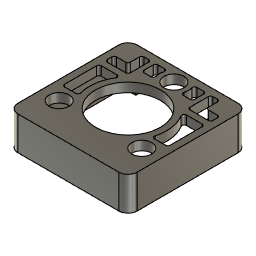
Laser Shroud (Autodesk Fusion 360 design; units mm, degrees)
Autodesk Fusion 360 part; units mm, degrees
sketch "Sketch1" plane through (0, 0, 0) normal (0, 0, 1) x (1, 0, 0) in component "Laser Shroud Mount"
  line L0 (0, 0) -> (39, 0)
  line L1 (39, 0) -> (39, 39)
  line L2 (39, 39) -> (0, 39)
  line L3 (0, 39) -> (0, 0)
  dimension "d1" = 39
  dimension "d2" = 39
  constraint horizontal L0
  constraint vertical L1
  constraint horizontal L2
  constraint vertical L3
  constraint coincident L0.start L3.end
  measures "d1" distance of L0.start L0.end
  measures "d2" distance of L0.start L2.end
extrude "Extrude1" add sketch "Sketch1" along normal blind 3 in component "Laser Shroud Mount"
sketch "Sketch2" plane through (0, 0, 3) normal (0, 0, 1) x (-1, 0, 0) in component "Laser Shroud Mount"
  line L0 (0, -39) -> (0, 0)
  line L1 (0, 0) -> (-39, 0)
  line L2 (-39, 0) -> (-39, -39)
  line L3 (-39, -39) -> (0, -39)
  line L4 (-19.5, -39) -> (-19.5, 0) construction
  line L5 (0, -19.5) -> (-39, -19.5) construction
  circle A0 centre (-19.5, -19.5) radius 10.6
  line L6 (-35, -35) -> (-4, -35) construction
  line L7 (-4, -35) -> (-4, -4) construction
  line L8 (-4, -4) -> (-35, -4) construction
  line L9 (-35, -4) -> (-35, -35) construction
  line L10 (-35, -35) -> (-4, -4) construction
  line L11 (-4, -35) -> (-35, -4) construction
  circle A1 centre (-4, -35) radius 1.75
  circle A2 centre (-35, -35) radius 1.75
  circle A3 centre (-4, -4) radius 1.75
  circle A4 centre (-35, -4) radius 1.75
  point P0 (-19.5, -19.5)
  dimension "d5" = 21.2
  dimension "d6" = 31
  dimension "d7" = 31
  dimension "d8" = 3.5
  dimension "d9" = 3.5
  dimension "d10" = 3.5
  dimension "d11" = 3.5
  constraint midpoint L3 L4.start
  constraint midpoint L1 L4.end
  constraint midpoint L0 L5.start
  constraint midpoint L2 L5.end
  constraint midpoint L5 P0
  constraint horizontal L6
  constraint perpendicular L6 L7
  constraint parallel L6 L8
  constraint parallel L7 L9
  constraint coincident L10 P0
  constraint coincident L11 P0
  constraint coincident P0 A0.centre
  constraint coincident L6.end L7.start
  constraint coincident L6.start L9.end
  constraint coincident L7.end L8.start
  constraint coincident L8.end L9.start
  measures "d5" diameter of A0
  measures "d6" distance of L7.end L8.end
  measures "d7" distance of L6.end L7.end
  measures "d8" diameter of A1
  measures "d9" diameter of A2
  measures "d10" diameter of A3
  measures "d11" diameter of A4
extrude "Extrude2" cut sketch "Sketch2" against normal up to surface (3 mm away) contours A0 in component "Laser Shroud Mount"
sketch "Sketch3" plane through (0, 0, 3) normal (0, 0, 1) x (-1, 0, 0) in component "Laser Shroud Mount"
  circle A0 centre (-19.5, -19.5) radius 10.6
  line L0 (0, -39) -> (0, 0)
  line L1 (0, 0) -> (-39, 0)
  line L2 (-39, 0) -> (-39, -39)
  line L3 (-39, -39) -> (0, -39)
  line L4 (-19.5, -39) -> (-19.5, 0) construction
  line L5 (0, -34.5) -> (-39, -34.5) construction
  circle A1 centre (-19.5, -34.5) radius 3.25
  line L6 (0, -10.5) -> (-39, -10.5) construction
  line L7 (-6, -39) -> (-6, 0) construction
  circle A2 centre (-6, -10.5) radius 3.25
  line L8 (-33, -39) -> (-33, 0) construction
  circle A3 centre (-33, -10.5) radius 3.25
  dimension "d14" = 4.5
  dimension "d15" = 6.5
  dimension "d16" = 6.5
  dimension "d18" = 10.5
  dimension "d19" = 6
  dimension "d21" = 6
  dimension "d22" = 6.5
  constraint midpoint L3 L4.start
  constraint midpoint L1 L4.end
  constraint coincident L0 L5.start
  constraint coincident L2 L5.end
  constraint perpendicular L2 L5
  constraint midpoint L5 A1.centre
  constraint coincident L0 L6.start
  constraint coincident L2 L6.end
  constraint perpendicular L2 L6
  constraint coincident L1 L7.end
  constraint perpendicular L1 L7
  constraint coincident L7 A2.centre
  constraint coincident L6 A2.centre
  constraint coincident L3 L8.start
  constraint coincident L1 L8.end
  constraint perpendicular L1 L8
  constraint coincident L8 A3.centre
  constraint coincident L6 A3.centre
  measures "d14" distance of L3 L5
  measures "d15" diameter of A1
  measures "d16" diameter of A2
  measures "d18" distance of L1 L6
  measures "d19" distance of L0 L7
  measures "d21" distance of L2 L8
  measures "d22" diameter of A3
extrude "Extrude3" cut sketch "Sketch3" against normal blind 3.2 contours A1 | A2 | A3 in component "Laser Shroud Mount"
sketch "Sketch4" plane through (0, 0, 3) normal (0, 0, 1) x (-1, 0, 0) in component "Laser Shroud Mount"
  circle A0 centre (-19.5, -34.5) radius 3.25 construction
  circle A1 centre (-6, -10.5) radius 3.25
  circle A2 centre (-33, -10.5) radius 3.25
  circle A3 centre (-19.5, -19.5) radius 10.6
  line L0 (0, -39) -> (0, 0)
  line L1 (0, 0) -> (-39, 0)
  line L2 (-39, 0) -> (-39, -39)
  line L3 (-39, -39) -> (0, -39)
  line L4 (0, -36.75) -> (-39, -36.75) construction
  line L5 (-6.75, -39) -> (-6.75, 0) construction
  line L6 (-32.25, -39) -> (-32.25, 0) construction
  line L7 (0, -32.25) -> (-39, -32.25) construction
  line L8 (-6.75, -36.75) -> (-6.75, -32.25)
  line L9 (-2.25, -39) -> (-2.25, 0) construction
  line L10 (-6.75, -32.25) -> (-2.25, -32.25)
  line L11 (-2.25, -32.25) -> (-2.25, -29.25)
  line L12 (0, -19.5) -> (-39, -19.5) construction
  line L13 (-19.5, -39) -> (-19.5, 0) construction
  line L14 (-6.75, -36.75) -> (-9.75, -36.75)
  line L15 (-2.25, -29.25) -> (-9.75, -29.25)
  line L16 (-9.75, -29.25) -> (-9.75, -36.75)
  line L17 (-11.25, -36.75) -> (-11.25, -32.25)
  line L18 (-11.25, -36.75) -> (-15.3167, -36.75)
  line L19 (-11.25, -32.25) -> (-15.3167, -32.25)
  line L20 (-2.25, -27.25) -> (-9.5653, -27.25)
  line L21 (-2.25, -15.25) -> (-7.6384, -15.25)
  line L22 (-2.25, -27.25) -> (-2.25, -15.25)
  line L23 (0, -2) -> (-39, -2) construction
  arc A4 (-9.5653, -27.25) -> (-7.6384, -15.25) centre (-19.5, -19.5) ccw
  arc A5 (-15.3167, -36.75) -> (-15.3167, -32.25) centre (-19.5, -34.5) ccw
  arc A6 (-31.3616, -15.25) -> (-29.4347, -27.25) centre (-19.5, -19.5) ccw
  line L24 (-36.75, -15.25) -> (-31.3616, -15.25)
  line L25 (-36.75, -27.25) -> (-36.75, -15.25)
  line L26 (-36.75, -27.25) -> (-29.4347, -27.25)
  line L27 (-36.75, -29.25) -> (-29.25, -29.25)
  line L28 (-36.75, -32.25) -> (-36.75, -29.25)
  line L29 (-29.25, -29.25) -> (-29.25, -36.75)
  line L30 (-32.25, -32.25) -> (-36.75, -32.25)
  line L31 (-32.25, -36.75) -> (-32.25, -32.25)
  line L32 (-32.25, -36.75) -> (-29.25, -36.75)
  line L33 (-27.75, -36.75) -> (-27.75, -32.25)
  arc A7 (-23.6833, -32.25) -> (-23.6833, -36.75) centre (-19.5, -34.5) ccw
  line L34 (-27.75, -32.25) -> (-23.6833, -32.25)
  line L35 (-27.75, -36.75) -> (-23.6833, -36.75)
  dimension "d25" = 2.25
  dimension "d26" = 6.75
  dimension "d27" = 6.75
  dimension "d28" = 6.75
  dimension "d29" = 3
  dimension "d34" = 3
  dimension "d35" = 1.5
  dimension "d36" = 2
  dimension "d37" = 12
  dimension "d38" = 2
  constraint coincident L0 L4.start
  constraint coincident L2 L4.end
  constraint perpendicular L2 L4
  constraint coincident L3 L5.start
  constraint coincident L1 L5.end
  constraint perpendicular L1 L5
  constraint coincident L3 L6.start
  constraint coincident L1 L6.end
  constraint perpendicular L1 L6
  constraint coincident L0 L7.start
  constraint coincident L2 L7.end
  constraint perpendicular L2 L7
  constraint coincident L4 L8.start
  constraint coincident L5 L8.start
  constraint coincident L5 L8.end
  constraint coincident L7 L8.end
  constraint perpendicular L7 L8
  constraint coincident L3 L9.start
  constraint coincident L1 L9.end
  constraint perpendicular L1 L9
  constraint coincident L9 L10.end
  constraint coincident L7 L10.end
  constraint perpendicular L7 L11
  constraint midpoint L0 L12.start
  constraint midpoint L2 L12.end
  constraint midpoint L3 L13.start
  constraint midpoint L1 L13.end
  constraint perpendicular L8 L14
  constraint perpendicular L11 L15
  constraint perpendicular L4 L16
  constraint coincident L4 L17.start
  constraint coincident L7 L17.end
  constraint perpendicular L7 L17
  constraint coincident L4 L18.end
  constraint coincident L7 L19.end
  constraint coincident L9 L20.start
  constraint perpendicular L9 L20
  constraint coincident L9 L21.start
  constraint perpendicular L5 L21
  constraint coincident L0 L23.start
  constraint coincident L2 L23.end
  constraint perpendicular L2 L23
  constraint concentric A3 A4
  constraint symmetric L8.start L13 L31.start
  constraint symmetric L8.end L13 L30.start
  constraint symmetric L10.end L13 L28.start
  constraint symmetric L11.end L13 L27.start
  constraint symmetric L13 L14.end L29.end
  constraint symmetric L13 L15.end L27.end
  constraint symmetric L13 L17.start L33.start
  constraint symmetric L13 L17.end L33.end
  constraint symmetric L13 L18.end A7.end
  constraint symmetric L13 L19.end A7.start
  constraint symmetric L13 L20.start L25.start
  constraint symmetric L13 L20.end A6.end
  constraint symmetric L13 L21.start L24.start
  constraint symmetric L13 L21.end A6.start
  constraint symmetric L13 A4 A6
  constraint symmetric L13 A5 A7
  measures "d25" distance of L3 L4
  measures "d26" distance of L0 L5
  measures "d27" distance of L2 L6
  measures "d28" distance of L3 L7
  measures "d29" distance of L10.end L11.end
  measures "d34" distance of L8.start L14.end
  measures "d35" distance of L16 L17
  measures "d36" distance of L15 L20
  measures "d37" distance of L20 L21
  measures "d38" distance of L1 L23
extrude "Extrude4" cut sketch "Sketch4" against normal up to surface (3 mm away) contours L8 L10 L11 L14 L15 L16 | L17 L18 L19 A5 | L20 L21 L22 A4 | A6 L24 L25 L26 | L27 L28 L29 L30 L31 L32 | L33 A7 L34 L35 in component "Laser Shroud Mount"
fillet "Fillet1" radius 3 4 edges at (0, 39, 1.5) (0, 0, 1.5) (39, 0, 1.5) (39, 39, 1.5) in component "Laser Shroud Mount"
fillet "Fillet3" radius 0.75 4 edges at (11.25, 36.75, 1.5) (11.25, 32.25, 1.5) (15.3167, 32.25, 1.5) (15.3167, 36.75, 1.5) in component "Laser Shroud Mount"
fillet "Fillet3" radius 0.75 4 edges at (23.6833, 36.75, 1.5) (23.6833, 32.25, 1.5) (27.75, 36.75, 1.5) (27.75, 32.25, 1.5) in component "Laser Shroud Mount"
fillet "Fillet3" radius 0.75 6 edges at (29.25, 36.75, 1.5) (32.25, 36.75, 1.5) (32.25, 32.25, 1.5) (36.75, 32.25, 1.5) (36.75, 29.25, 1.5) (29.25, 29.25, 1.5) in component "Laser Shroud Mount"
fillet "Fillet3" radius 0.75 6 edges at (6.75, 36.75, 1.5) (6.75, 32.25, 1.5) (2.25, 32.25, 1.5) (2.25, 29.25, 1.5) (9.75, 29.25, 1.5) (9.75, 36.75, 1.5) in component "Laser Shroud Mount"
fillet "Fillet3" radius 0.75 4 edges at (29.4347, 27.25, 1.5) (36.75, 27.25, 1.5) (36.75, 15.25, 1.5) (31.3616, 15.25, 1.5) in component "Laser Shroud Mount"
fillet "Fillet3" radius 0.75 4 edges at (2.25, 27.25, 1.5) (9.5653, 27.25, 1.5) (7.6384, 15.25, 1.5) (2.25, 15.25, 1.5) in component "Laser Shroud Mount"
sketch "Sketch1 (2)" plane through (0, 0, 0) normal (0, 0, -1) x (1, 0, 0)
  arc A0 (6.75, -33) -> (6, -32.25) centre (6, -33) ccw
  line L0 (6, -32.25) -> (3, -32.25)
  arc A1 (2.25, -31.5) -> (3, -32.25) centre (3, -31.5) ccw
  line L1 (2.25, -31.5) -> (2.25, -30)
  arc A2 (3, -29.25) -> (2.25, -30) centre (3, -30) ccw
  line L2 (3, -29.25) -> (9, -29.25)
  arc A3 (9.75, -30) -> (9, -29.25) centre (9, -30) ccw
  line L3 (9.75, -30) -> (9.75, -36)
  arc A4 (9, -36.75) -> (9.75, -36) centre (9, -36) ccw
  line L4 (9, -36.75) -> (7.5, -36.75)
  arc A5 (6.75, -36) -> (7.5, -36.75) centre (7.5, -36) ccw
  line L5 (6.75, -36) -> (6.75, -33)
  arc A6 (33, -32.25) -> (32.25, -33) centre (33, -33) ccw
  line L6 (32.25, -33) -> (32.25, -36)
  arc A7 (31.5, -36.75) -> (32.25, -36) centre (31.5, -36) ccw
  line L7 (31.5, -36.75) -> (30, -36.75)
  arc A8 (29.25, -36) -> (30, -36.75) centre (30, -36) ccw
  line L8 (29.25, -36) -> (29.25, -30)
  arc A9 (30, -29.25) -> (29.25, -30) centre (30, -30) ccw
  line L9 (30, -29.25) -> (36, -29.25)
  arc A10 (36.75, -30) -> (36, -29.25) centre (36, -30) ccw
  line L10 (36.75, -30) -> (36.75, -31.5)
  arc A11 (36, -32.25) -> (36.75, -31.5) centre (36, -31.5) ccw
  line L11 (36, -32.25) -> (33, -32.25)
  arc A12 (36, -39) -> (39, -36) centre (36, -36) ccw
  line L12 (39, -36) -> (39, -3)
  arc A13 (39, -3) -> (36, 0) centre (36, -3) ccw
  line L13 (36, 0) -> (3, 0)
  arc A14 (3, 0) -> (0, -3) centre (3, -3) ccw
  line L14 (0, -3) -> (0, -36)
  arc A15 (0, -36) -> (3, -39) centre (3, -36) ccw
  line L15 (3, -39) -> (36, -39)
  line L16 (32.383, -15.25) -> (36, -15.25)
  arc A16 (36.75, -16) -> (36, -15.25) centre (36, -16) ccw
  line L17 (36.75, -16) -> (36.75, -26.5)
  arc A17 (36, -27.25) -> (36.75, -26.5) centre (36, -26.5) ccw
  line L18 (36, -27.25) -> (30.8676, -27.25)
  arc A18 (30.229, -26.1067) -> (30.8676, -27.25) centre (30.8676, -26.5) ccw
  arc A19 (30.229, -26.1067) -> (31.6593, -16.1966) centre (19.5, -19.5) ccw
  arc A20 (32.383, -15.25) -> (31.6593, -16.1966) centre (32.383, -16) ccw
  line L19 (14.2085, -36.75) -> (12, -36.75)
  arc A21 (11.25, -36) -> (12, -36.75) centre (12, -36) ccw
  line L20 (11.25, -36) -> (11.25, -33)
  arc A22 (12, -32.25) -> (11.25, -33) centre (12, -33) ccw
  line L21 (12, -32.25) -> (14.2085, -32.25)
  arc A23 (14.9301, -33.2045) -> (14.2085, -32.25) centre (14.2085, -33) ccw
  arc A24 (14.9301, -33.2045) -> (14.9301, -35.7955) centre (19.5, -34.5) ccw
  arc A25 (14.2085, -36.75) -> (14.9301, -35.7955) centre (14.2085, -36) ccw
  line L22 (8.1324, -27.25) -> (3, -27.25)
  arc A26 (2.25, -26.5) -> (3, -27.25) centre (3, -26.5) ccw
  line L23 (2.25, -26.5) -> (2.25, -16)
  arc A27 (3, -15.25) -> (2.25, -16) centre (3, -16) ccw
  line L24 (3, -15.25) -> (6.617, -15.25)
  arc A28 (7.3407, -16.1966) -> (6.617, -15.25) centre (6.617, -16) ccw
  arc A29 (7.3407, -16.1966) -> (8.771, -26.1067) centre (19.5, -19.5) ccw
  arc A30 (8.1324, -27.25) -> (8.771, -26.1067) centre (8.1324, -26.5) ccw
  line L25 (24.7915, -32.25) -> (27, -32.25)
  arc A31 (27.75, -33) -> (27, -32.25) centre (27, -33) ccw
  line L26 (27.75, -33) -> (27.75, -36)
  arc A32 (27, -36.75) -> (27.75, -36) centre (27, -36) ccw
  line L27 (27, -36.75) -> (24.7915, -36.75)
  arc A33 (24.0699, -35.7955) -> (24.7915, -36.75) centre (24.7915, -36) ccw
  arc A34 (24.0699, -35.7955) -> (24.0699, -33.2045) centre (19.5, -34.5) ccw
  arc A35 (24.7915, -32.25) -> (24.0699, -33.2045) centre (24.7915, -33) ccw
  circle A36 centre (19.5, -19.5) radius 10.6
  line L28 (37, -36) -> (37, -3)
  arc A37 (37, -3) -> (36, -2) centre (36, -3) ccw
  line L29 (36, -2) -> (3, -2)
  arc A38 (3, -2) -> (2, -3) centre (3, -3) ccw
  line L30 (2, -3) -> (2, -36)
  arc A39 (2, -36) -> (3, -37) centre (3, -36) ccw
  line L31 (3, -37) -> (36, -37)
  arc A40 (36, -37) -> (37, -36) centre (36, -36) ccw
  line L32 (39, -36) -> (39, -3)
  arc A41 (39, -3) -> (36, 0) centre (36, -3) ccw
  line L33 (36, 0) -> (3, 0)
  arc A42 (3, 0) -> (0, -3) centre (3, -3) ccw
  line L34 (0, -3) -> (0, -36)
  arc A43 (0, -36) -> (3, -39) centre (3, -36) ccw
  line L35 (3, -39) -> (36, -39)
  arc A44 (36, -39) -> (39, -36) centre (36, -36) ccw
  circle A45 centre (19.5, -34.5) radius 3.25
  circle A46 centre (6, -10.5) radius 3.25
  circle A47 centre (33, -10.5) radius 3.25
  dimension "d63" = -2
  dimension "d64" = 0
  measures "d64" distance of L12
extrude "Extrude5" add sketch "Sketch1 (2)" along normal blind 8 contours A12 L12 A13 L13 A14 L14 A15 L15 L32 A41 L33 A42 L34 A43 L35 A44 | L31 A45 picked at (18.9296, -37.0877) in component "Laser Shroud Mount"
sketch "Sketch2 (2)" plane through (0, 37, 0) normal (0, -1, 0) x (1, 0, 0)
  line L0 (36, 0) -> (21.5767, 0)
  line L1 (21.5767, 0) -> (17.4233, 0)
  line L2 (17.4233, 0) -> (3, 0)
  line L3 (3, 0) -> (3, -8)
  line L4 (3, -8) -> (36, -8)
  line L5 (36, -8) -> (36, 0)
  line L6 (19.5, 0) -> (19.5, -8) construction
  line L7 (4.5, -8) -> (34.5, -8)
  line L8 (34.5, -8) -> (34.5, -1)
  line L9 (34.5, -1) -> (4.5, -1)
  line L10 (4.5, -1) -> (4.5, -8)
  dimension "d67" = 30
  dimension "d68" = 7
  dimension "d69" = 1.5
  constraint midpoint L1 L6.start
  constraint midpoint L4 L6.end
  constraint horizontal L7
  constraint vertical L8
  constraint horizontal L9
  constraint vertical L10
  constraint coincident L4 L7.start
  measures "d67" distance of L7.start L7.end
  measures "d68" distance of L7.start L9.end
  measures "d69" distance of L3 L10
extrude "Extrude6" cut sketch "Sketch2 (2)" against normal up to surface (2 mm away) contours L4 L7 L8 L9 L10 in component "Laser Shroud Mount"
sketch "Sketch3 (2)" plane through (0, 0, 0) normal (0, 0, -1) x (1, 0, 0)
  line L0 (3, -37) -> (17.4233, -37)
  arc A0 (21.5767, -37) -> (17.4233, -37) centre (19.5, -34.5) ccw
  line L1 (21.5767, -37) -> (36, -37)
  arc A1 (36, -37) -> (37, -36) centre (36, -36) ccw
  line L2 (37, -36) -> (37, -3)
  arc A2 (37, -3) -> (36, -2) centre (36, -3) ccw
  line L3 (36, -2) -> (3, -2)
  arc A3 (3, -2) -> (2, -3) centre (3, -3) ccw
  line L4 (2, -3) -> (2, -36)
  arc A4 (2, -36) -> (3, -37) centre (3, -36) ccw
  arc A5 (6.75, -33) -> (6, -32.25) centre (6, -33) ccw
  line L5 (6, -32.25) -> (3, -32.25)
  arc A6 (2.25, -31.5) -> (3, -32.25) centre (3, -31.5) ccw
  line L6 (2.25, -31.5) -> (2.25, -30)
  arc A7 (3, -29.25) -> (2.25, -30) centre (3, -30) ccw
  line L7 (3, -29.25) -> (9, -29.25)
  arc A8 (9.75, -30) -> (9, -29.25) centre (9, -30) ccw
  line L8 (9.75, -30) -> (9.75, -36)
  arc A9 (9, -36.75) -> (9.75, -36) centre (9, -36) ccw
  line L9 (9, -36.75) -> (7.5, -36.75)
  arc A10 (6.75, -36) -> (7.5, -36.75) centre (7.5, -36) ccw
  line L10 (6.75, -36) -> (6.75, -33)
  arc A11 (33, -32.25) -> (32.25, -33) centre (33, -33) ccw
  line L11 (32.25, -33) -> (32.25, -36)
  arc A12 (31.5, -36.75) -> (32.25, -36) centre (31.5, -36) ccw
  line L12 (31.5, -36.75) -> (30, -36.75)
  arc A13 (29.25, -36) -> (30, -36.75) centre (30, -36) ccw
  line L13 (29.25, -36) -> (29.25, -30)
  arc A14 (30, -29.25) -> (29.25, -30) centre (30, -30) ccw
  line L14 (30, -29.25) -> (36, -29.25)
  arc A15 (36.75, -30) -> (36, -29.25) centre (36, -30) ccw
  line L15 (36.75, -30) -> (36.75, -31.5)
  arc A16 (36, -32.25) -> (36.75, -31.5) centre (36, -31.5) ccw
  line L16 (36, -32.25) -> (33, -32.25)
  line L17 (32.383, -15.25) -> (36, -15.25)
  arc A17 (36.75, -16) -> (36, -15.25) centre (36, -16) ccw
  line L18 (36.75, -16) -> (36.75, -26.5)
  arc A18 (36, -27.25) -> (36.75, -26.5) centre (36, -26.5) ccw
  line L19 (36, -27.25) -> (30.8676, -27.25)
  arc A19 (30.229, -26.1067) -> (30.8676, -27.25) centre (30.8676, -26.5) ccw
  arc A20 (30.229, -26.1067) -> (31.6593, -16.1966) centre (19.5, -19.5) ccw
  arc A21 (32.383, -15.25) -> (31.6593, -16.1966) centre (32.383, -16) ccw
  line L20 (14.2085, -36.75) -> (12, -36.75)
  arc A22 (11.25, -36) -> (12, -36.75) centre (12, -36) ccw
  line L21 (11.25, -36) -> (11.25, -33)
  arc A23 (12, -32.25) -> (11.25, -33) centre (12, -33) ccw
  line L22 (12, -32.25) -> (14.2085, -32.25)
  arc A24 (14.9301, -33.2045) -> (14.2085, -32.25) centre (14.2085, -33) ccw
  arc A25 (14.9301, -33.2045) -> (14.9301, -35.7955) centre (19.5, -34.5) ccw
  arc A26 (14.2085, -36.75) -> (14.9301, -35.7955) centre (14.2085, -36) ccw
  line L23 (8.1324, -27.25) -> (3, -27.25)
  arc A27 (2.25, -26.5) -> (3, -27.25) centre (3, -26.5) ccw
  line L24 (2.25, -26.5) -> (2.25, -16)
  arc A28 (3, -15.25) -> (2.25, -16) centre (3, -16) ccw
  line L25 (3, -15.25) -> (6.617, -15.25)
  arc A29 (7.3407, -16.1966) -> (6.617, -15.25) centre (6.617, -16) ccw
  arc A30 (7.3407, -16.1966) -> (8.771, -26.1067) centre (19.5, -19.5) ccw
  arc A31 (8.1324, -27.25) -> (8.771, -26.1067) centre (8.1324, -26.5) ccw
  line L26 (24.7915, -32.25) -> (27, -32.25)
  arc A32 (27.75, -33) -> (27, -32.25) centre (27, -33) ccw
  line L27 (27.75, -33) -> (27.75, -36)
  arc A33 (27, -36.75) -> (27.75, -36) centre (27, -36) ccw
  line L28 (27, -36.75) -> (24.7915, -36.75)
  arc A34 (24.0699, -35.7955) -> (24.7915, -36.75) centre (24.7915, -36) ccw
  arc A35 (24.0699, -35.7955) -> (24.0699, -33.2045) centre (19.5, -34.5) ccw
  arc A36 (24.7915, -32.25) -> (24.0699, -33.2045) centre (24.7915, -33) ccw
  circle A37 centre (6, -10.5) radius 3.25
  circle A38 centre (33, -10.5) radius 3.25
  circle A39 centre (19.5, -19.5) radius 10.6
  line L29 (21.5767, -37) -> (36, -37)
  line L30 (4.5, -37) -> (34.5, -37)
  line L31 (34.5, -37) -> (34.5, -36.4)
  line L32 (34.5, -36.4) -> (33, -36.4)
  line L33 (19.5, -37) -> (19.5, -2) construction
  line L34 (4.5, -37) -> (4.5, -36.4)
  line L35 (4.5, -36.4) -> (6, -36.4)
  line L36 (33, -35.5) -> (33, -36.4)
  line L37 (6, -35.5) -> (6, -36.4)
  line L38 (3, -37) -> (4.5, -37)
  line L39 (34.5, -37) -> (36, -37)
  arc A40 (2, -36) -> (3, -37) centre (3, -36) ccw
  line L40 (6, -35.5) -> (2, -35.5)
  line L41 (2, -35.5) -> (2, -36)
  arc A41 (36, -37) -> (37, -36) centre (36, -36) ccw
  arc A42 (36, -37) -> (37, -36) centre (36, -36) ccw
  line L42 (33, -35.5) -> (37, -35.5)
  line L43 (37, -35.5) -> (37, -36)
  dimension "d74" = 0.6
  dimension "d90" = 0
  dimension "d91" = 0
  constraint coincident L30.end L31.start
  constraint perpendicular L1 L31
  constraint perpendicular L31 L32
  constraint midpoint L30 L33.start
  constraint midpoint L3 L33.end
  constraint symmetric L30.end L33 L30.start
  constraint symmetric L31.end L33 L34.end
  constraint symmetric L32.end L33 L35.end
  constraint perpendicular L32 L36
  constraint perpendicular L35 L37
  constraint coincident L0.start A4.end
  constraint coincident L30.start L34.start
  constraint coincident L1.end A1.start
  constraint coincident L4 L40.end
  constraint perpendicular L4 L40
  constraint coincident L4.end A4.start
  constraint coincident L2 L42.end
  constraint perpendicular L2 L42
  constraint coincident A1.end L2.start
  measures "d74" distance of L30.end L31.end
extrude "Extrude7" add sketch "Sketch3 (2)" along normal up to surface (8 mm away) contours L0 L4 A4 L34 L35 L37 L38 A40 L40 L41 | L1 A1 L2 L29 L31 L32 L36 L39 A41 A42 L42 L43 in component "Laser Shroud Mount"
fillet "Fillet5" radius 1 2 edges at (2, 35.5, -4) (37, 35.5, -4) in component "Laser Shroud Mount"
sketch "Sketch6" plane through (0, 0, -1) normal (0, 0, -1) x (1, 0, 0)
  line L0 (4.5, -39) -> (34.5, -39)
  line L1 (34.5, -39) -> (34.5, -37)
  line L2 (34.5, -37) -> (4.5, -37)
  line L3 (4.5, -37) -> (4.5, -39)
  line L4 (34.5, -39) -> (4.5, -39)
  line L5 (4.5, -39) -> (4.5, -37)
  line L6 (4.5, -37) -> (34.5, -37)
  line L7 (34.5, -37) -> (34.5, -39)
  constraint horizontal L4
  constraint vertical L5
  constraint horizontal L6
  constraint vertical L7
  constraint coincident L2.end L3.start
  constraint coincident L0.end L1.start
extrude "Extrude10" cut sketch "Sketch6" against normal up to surface (1 mm away) in component "Laser Shroud Mount"
component "Laser Shroud Mount" placed x (1, 0, 0) y (0, 1, 0) z (0, 0, 1) at (0, 0, 0)
named bodies: "Laser Shroud"
